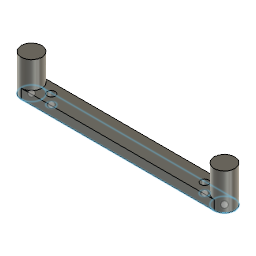
Suport waveshare (Autodesk Fusion 360 design; units mm, degrees)
part number: 2026-03-13-09-46-56-234
Autodesk Fusion 360 part; units mm, degrees
sketch "Boceto1" plane through (0, 0, 0) normal (0, 0, 1) x (1, 0, 0)
  line L0 (3.25, 0) -> (64.25, 0)
  line L1 (64.25, 6.5) -> (3.25, 6.5)
  circle A0 centre (9.5, 3.25) radius 1.25
  circle A1 centre (3.25, 3.25) radius 3.25
  circle A2 centre (64.25, 3.25) radius 3.25
  circle A3 centre (58, 3.25) radius 1.25
  dimension "d12" = 2.5
  dimension "d14" = 6.5
  constraint horizontal L0
  constraint horizontal L1
  constraint coincident A1 L1.end
  constraint coincident A1 L0.start
  constraint coincident A2 L1.start
  constraint coincident A2 L0.end
  measures "d12" diameter of A0
  measures "d14" diameter of A1
extrude "Extruir1" add sketch "Boceto1" along normal blind 3 contours L0 L1 A1 A2
extrude "Extruir2" add sketch "Boceto1" along normal blind 10.5 contours A1
extrude "Extruir3" add sketch "Boceto1" along normal blind 10.5 contours A2
extrude "Extruir4" add 1 faces at (3.7107, 2.452, 10.5) along direction (0, 0, 1) blind 1
extrude "Extruir5" add 1 faces at (63.0857, 4.3303, 10.5) along direction (0, 0, 1) blind 1
